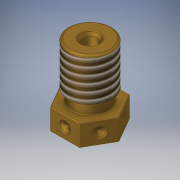
# Autodesk Inventor part: Nozzle
Saved by Autodesk Inventor 2019 (Build 230136000, 136)
## iProperties
Created: 2021-03-14
Part Number: Nozzle
Material: Générique
Document SubType Name: Modeling
Designer: thoma
Density: 1 g/cm^3
Appearance: Laiton - Satiné
Author: thoma
Autodesk Inventor part; units mm, degrees
ref_plane "YZ Plane" through (0, 0, 0) normal (1, 0, 0) x (0, 1, 0)
ref_plane "XZ Plane" through (0, 0, 0) normal (0, 1, 0) x (-1, 0, 0)
ref_plane "XY Plane" through (0, 0, 0) normal (0, 0, 1) x (1, 0, 0)
sketch "Esquisse1" plane through (0, 0, 0) normal (0, 0, 1) x (1, 0, 0)
  line L0 (0, 0) -> (3, 0)
  line L1 (3, 0) -> (3, -6)
  line L2 (3, -6) -> (2.5, -6)
  line L3 (2.5, -6) -> (2.5, -7.5)
  line L4 (2.5, -7.5) -> (3.5, -7.5)
  line L5 (3.5, -7.5) -> (3.5, -10.5)
  line L6 (0, 0) -> (0, -12.5)
  line L7 (0, -12.5) -> (0.8402, -11.0448) construction
  line L8 (0, -12.5) -> (1.6804, -12.5) construction
  line L9 (0, -12.5) -> (0.5, -12.5)
  line L10 (0.5, -12.5) -> (1.6547, -10.5)
  line L11 (3.5, -10.5) -> (1.6547, -10.5)
  dimension "d0" = 3
  dimension "d1" = 6
  dimension "d2" = 0.5
  dimension "d3" = 1.5
  dimension "d4" = 1
  dimension "d5" = 3
  dimension "d7" = 12.5
  dimension "d8" = 60
  dimension "d9" = 0.5
  constraints: 24 end point, 4 perpendicular, 3 horizontal, 2 vertical, 1 equal length, 1 parallel, 1 point on line
  measures "d0" distance of L0.start L0.end
  measures "d1" distance of L0.end L1.end
  measures "d2" distance of L1.end L2.end
  measures "d3" distance of L2.end L3.end
  measures "d4" distance of L3.end L4.end
  measures "d5" distance of L4.end L5.end
  measures "d7" distance of L0.start L6.end
  measures "d8" angle of L8 L7
  measures "d9" distance of L6.end L9.end
revolve "Révolution1" add sketch "Esquisse1" angle 360 about axis through (0, 0, 0) along (0, -1, 0)
sketch "Esquisse3" plane through (0, 0, 0) normal (0, 1, 0) x (1, 0, 0)
  circle A0 centre (0, 0) radius 3.5 projected
  line L0 (2.0207, 3.5) -> (4.0415, 0)
  line L1 (4.0415, 0) -> (2.0207, -3.5)
  line L2 (2.0207, -3.5) -> (-2.0207, -3.5)
  line L3 (-2.0207, -3.5) -> (-4.0415, 0)
  line L4 (-4.0415, 0) -> (-2.0207, 3.5)
  line L5 (-2.0207, 3.5) -> (2.0207, 3.5)
  point P0 (0, 3.5)
  dimension "d11" = 7
  constraints: 12 end point, 1 coincident, 1 midpoint, 1 vertical alignment, 14 other
  measures "d11" distance between parallel lines of L2 L5
extrude "Extrusion1" add sketch "Esquisse3" against normal up to surface (3 mm away) from surface at -7.5 contours A0 L0 L1 | A0 L5 L0 | L1 L2 A0 | A0 L4 L5 | L2 L3 A0 | A0 L3 L4
sketch "Esquisse4" plane through (-4.0415, -10.5, 0) normal (-0.8660254, 0, -0.5) x (-0.5, 0, 0.8660254)
  circle A0 centre (-2.0207, 1.5) radius 0.75
  point P0 (-2.0207, 10.5)
  dimension "d14" = 1.5
  constraints: 1 centre point
  measures "d14" diameter of A0
extrude "Extrusion2" cut sketch "Esquisse4" against normal blind 0.5
chamfer "Chanfrein1" distance 0.4 distance2 0.75 1 edges at (-2.2213, -9, -2.1485) measured on face at (-2.3079, -9, -2.1985)
pattern_circular "Réseau circulaire1" count 6 over 360 about axis through (0, -6.75, 0) along (0, -1, 0) of "Extrusion2", "Chanfrein1"
sketch "Esquisse5" plane through (0, 0, 0) normal (0, 1, 0) x (1, 0, 0)
  circle A0 centre (0, 0) radius 0.5 projected
  circle A1 centre (0, 0) radius 1.3
  dimension "d23" = 2.6
  constraints: 1 centre point, 1 coincident
  measures "d23" diameter of A1
extrude "Extrusion3" cut sketch "Esquisse5" against normal blind 0.5 contours A0 | A1
sketch "Esquisse6" plane through (0, -0.5, 0) normal (0, 1, 0) x (1, 0, 0)
  circle A0 centre (0, 0) radius 0.5 projected
  circle A1 centre (0, 0) radius 1
  dimension "d26" = 2
  constraints: 1 centre point, 1 coincident
  measures "d26" diameter of A1
extrude "Extrusion4" cut sketch "Esquisse6" against normal up to surface (10 mm away) contours A0 | A1
sketch "Esquisse7" plane through (0, -12.5, 0) normal (0, -1, 0) x (1, 0, 0)
  circle A0 centre (0, 0) radius 1 projected
  circle A1 centre (0, 0) radius 0.2
  dimension "d29" = 0.4
  constraints: 1 centre point, 1 coincident
  measures "d29" diameter of A1
extrude "Extrusion5" cut sketch "Esquisse7" against normal up to next contours A1
chamfer "Chanfrein2" distance 0.4 distance2 0.3 1 edges at (-1.3, -0.5, 0) measured on face at (-1.3, -0.4, 0)
thread "Filetage1" size "M6x1" class "6g" standard "ANSI Metric M Profile" full length
chamfer "Chanfrein3" distance 0.2 distance2 0.3 1 edges at (-3, 0, 0) measured on face at (-3, -0.5, 0)
fillet "Congé1" radius 0.1 18 edges at (-1.3, -0.1001, 0) (-1.0001, -0.5, 0) (-2.5, -6, 0) (-2.5, -7.5, 0) (-1, -10.5, 0) (-1.6547, -10.5, 0) (3.3177, -9, -1.0494) (0.75, -9, -3.3979) (-2.5677, -9, -2.3485) (-3.3177, -9, 1.0494) (-0.75, -9, 3.3979) (2.5677, -9, 2.3485) (2.5964, -9, -1.4989) (0.0001, -9, -2.998) (-2.5963, -9, -1.4991) (-2.5964, -9, 1.4989) (-0.0001, -9, 2.998) (2.5963, -9, 1.4991)
fillet "Congé1" radius 0.1 32 edges at (-2.7, 0, 0) (-1.3, 0, 0) (-3, -0.2, 0) (-3, -6, 0) (-1, -0.5, 0) (3.0311, -7.5, -1.75) (0, -7.5, -3.5) (-3.0311, -7.5, -1.75) (-3.0311, -7.5, 1.75) (0, -7.5, 3.5) (3.0311, -7.5, 1.75) (-0.2, -10.5, 0) (4.0415, -9, 0) (3.0311, -10.5, -1.75) (2.0207, -9, -3.5) (3.4061, -9, -1.1005) (-2.0207, -9, -3.5) (0, -10.5, -3.5) (0.75, -9, -3.5) (-4.0415, -9, 0) (-3.0311, -10.5, -1.75) (-2.6561, -9, -2.3995) (-2.0207, -9, 3.5) (-3.0311, -10.5, 1.75) (-3.4061, -9, 1.1005) (2.0207, -9, 3.5) (0, -10.5, 3.5) (-0.75, -9, 3.5) (3.0311, -10.5, 1.75) (2.6561, -9, 2.3995) (-0.2, -12.5, 0) (-0.5, -12.5, 0)
